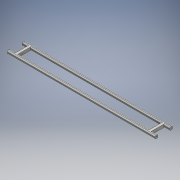
# Autodesk Inventor part: Desk foot holding bar
Saved by Autodesk Inventor 2016 (Build 200138000, 138)
## iProperties
Created: 2015-11-19
Part Number: Desk foot holding bar
Material: 常规
Document SubType Name: Modeling
Designer: Shawn Shi Feng
Density: 1 g/cm^3
Appearance: 默认
Author: Shawn Shi Feng
Autodesk Inventor part; units mm, degrees
ref_plane "YZ Plane" through (0, 0, 0) normal (1, 0, 0) x (0, 1, 0)
ref_plane "XZ Plane" through (0, 0, 0) normal (0, 1, 0) x (-1, 0, 0)
ref_plane "XY Plane" through (0, 0, 0) normal (0, 0, 1) x (1, 0, 0)
sketch "草图1" plane through (0, 0, 0) normal (0, 0, 1) x (1, 0, 0)
  line L0 (-326.5872, 86.4864) -> (428.4128, 86.4864)
  line L1 (428.4128, 86.4864) -> (428.4128, 71.4864)
  line L2 (-326.5872, 71.4864) -> (-326.5872, 86.4864)
  line L3 (428.4128, 11.4864) -> (428.4128, -3.5136)
  line L4 (428.4128, -3.5136) -> (-326.5872, -3.5136)
  line L5 (-326.5872, -3.5136) -> (-326.5872, 11.4864)
  line L6 (-284.5872, 71.4864) -> (-284.5872, 11.4864)
  line L7 (-296.5872, 11.4864) -> (-296.5872, 71.4864)
  line L8 (398.4128, 71.4864) -> (398.4128, 11.4864)
  line L9 (386.4128, 11.4864) -> (386.4128, 71.4864)
  line L10 (-296.5872, 71.4864) -> (-326.5872, 71.4864)
  line L11 (-326.5872, 11.4864) -> (-296.5872, 11.4864)
  line L12 (428.4128, 71.4864) -> (398.4128, 71.4864)
  line L13 (386.4128, 71.4864) -> (-284.5872, 71.4864)
  line L14 (-284.5872, 11.4864) -> (386.4128, 11.4864)
  line L15 (398.4128, 11.4864) -> (428.4128, 11.4864)
  point P0 (0, 0)
  point P1 (-326.5872, 78.9864)
  point P2 (-326.5872, 3.9864)
  dimension "d0" = 755
  dimension "d1" = 15
  dimension "d2" = 15
  dimension "d3" = 7.5
  dimension "d4" = 75
  dimension "d5" = 12
  dimension "d6" = 12
  dimension "d7" = 30
  dimension "d8" = 30
  constraints: 32 end point, 10 parallel, 4 horizontal, 4 perpendicular, 2 midpoint, 2 point on line
  measures "d0" distance of L0.start L0.end
  measures "d1" distance of L2.start L0.start
  measures "d2" distance of L4.end L5.end
  measures "d3" distance of L0.start point (-326.587, 78.986)
  measures "d4" distance of point (-326.587, 3.986) point (-326.587, 78.986)
  measures "d5" distance between parallel lines of L6 L7
  measures "d6" distance between parallel lines of L9 L8
  measures "d7" distance from line of L8 L1.end
  measures "d8" distance from line of L2.start L7
extrude "拉伸1" add sketch "草图1" along normal blind 15
fillet "圆角1" radius 5 1 edges at (50.9128, 86.4864, 15)
fillet "圆角2" radius 5 12 edges at (50.9128, 86.4864, 0) (50.9128, 71.4864, 15) (413.4128, 71.4864, 15) (413.4128, 11.4864, 15) (413.4128, 11.4864, 0) (50.9128, -3.5136, 15) (50.9128, 11.4864, 15) (50.9128, 11.4864, 0) (50.9128, -3.5136, 0) (-311.5872, 11.4864, 15) (-311.5872, 71.4864, 15) (-311.5872, 71.4864, 0)
fillet "圆角3" radius 5 3 edges at (-311.5872, 11.4864, 0) (413.4128, 71.4864, 0) (50.9128, 71.4864, 0)
sketch "草图2" plane through (428.4128, 76.4864, 15) normal (1, 0, 0) x (0, 0, -1)
  line L0 (15, 5) -> (15, 0) projected
  line L1 (10, -5) -> (5, -5) projected
  circle A0 centre (7.5, 2.5) radius 2.5
  circle A1 centre (7.5, -72.5) radius 2.5
  line L2 (15, -70) -> (15, -75) projected
  line L3 (10, -65) -> (5, -65) projected
  point P0 (15, -76.4864)
  dimension "d14" = 7.5
  dimension "d15" = 7.5
  dimension "d16" = 7.5
  dimension "d17" = 7.5
  dimension "d18" = 5
  constraints: 2 centre point, 1 coincident
  measures "d14" distance from line of L0 point (7.5, 2.5)
  measures "d15" distance from line of L1 point (7.5, 2.5)
  measures "d16" distance from line of L2 A1.centre
  measures "d17" distance from line of L3 A1.centre
  measures "d18" diameter of A1
extrude "拉伸2" cut sketch "草图2" against normal blind 800
